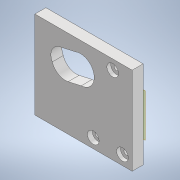
# Autodesk Inventor part: BOWDEN MOUNT
Saved by Autodesk Inventor 2020 (Build 240168000, 168)
## iProperties
Created: 2019-06-20
Part Number: BOWDEN MOUNT
Material: Generic
Document SubType Name: Modeling
Designer: pepd9
Density: 1 g/cm^3
Appearance: Default
Author: pepd9
Autodesk Inventor part; units mm, degrees
ref_plane "YZ Plane" through (0, 0, 0) normal (1, 0, 0) x (0, 1, 0)
ref_plane "XZ Plane" through (0, 0, 0) normal (0, 1, 0) x (-1, 0, 0)
ref_plane "XY Plane" through (0, 0, 0) normal (0, 0, 1) x (1, 0, 0)
ref_plane "Work Plane2" through (0, 0, 0) normal (0, 0, 1) x (1, 0, 0)
sketch "Sketch1" plane through (0, 0, 0) normal (0, 0, 1) x (1, 0, 0)
  line L0 (-10, 22.5) -> (10, 22.5)
  line L1 (10, 22.5) -> (10, -22.5)
  line L2 (10, -22.5) -> (-10, -22.5)
  line L3 (-10, -22.5) -> (-10, 22.5)
  circle A0 centre (0, 17.5) radius 1.25
  circle A1 centre (5, -17.5) radius 1.25
  point P0 (0, 0)
  dimension "d38" = 20
  dimension "d39" = 45
  dimension "d40" = 2.5
  dimension "d41" = 2.5
  dimension "d42" = 10
  dimension "d43" = 5
  dimension "d44" = 5
  dimension "d45" = 5
  constraints: 8 end point, 2 centre point, 2 parallel, 1 horizontal, 1 perpendicular
  measures "d38" distance of L0.start L0.end
  measures "d39" distance of L2.end L0.start
  measures "d40" diameter of A0
  measures "d41" diameter of A1
  measures "d42" distance from line of L1 A0.centre
  measures "d43" distance from line of L0 A0.centre
  measures "d44" distance from line of L2 A1.centre
  measures "d45" distance from line of L1 A1.centre
extrude "Extrusion1" add sketch "Sketch1" along normal blind 3.65 contours L0 L1 L2 L3 | A0 | A1
sketch "Sketch2" plane through (-10, 118.2358, 3.65) normal (-1, 0, 0) x (0, 0, 1)
  line L0 (-3.65, -95.7358) -> (-3.65, -140.7358) projected
  line L1 (-3.65, -140.7358) -> (0, -140.7358) projected
  line L2 (0, -95.7358) -> (0, -140.7358) projected
  line L3 (-3.65, -95.7358) -> (0, -95.7358) projected
  point P0 (-3.65, -118.2358)
extrude "Extrusion2" add sketch "Sketch2" along normal blind 30
sketch "Sketch3" plane through (0, 0, 3.65) normal (0, 0, 1) x (1, 0, 0)
  line L0 (10, -22.5) -> (10, 22.5) projected
  line L1 (10, 22.5) -> (-40, 22.5) projected
  line L2 (-40, -22.5) -> (-40, 22.5) projected
  line L3 (10, -22.5) -> (-40, -22.5) projected
  circle A0 centre (0, 17.5) radius 3 construction
  circle A1 centre (5, -17.5) radius 3 construction
  point P0 (0, 0)
  dimension "d48" = 6
  dimension "d49" = 6
  constraints: 2 centre point
  measures "d48" diameter of A0
  measures "d49" diameter of A1
extrude "Extrusion3" add sketch "Sketch3" along normal blind 2
ref_plane "Work Plane3" through (0, 0, 0) normal (0, 0, -1) x (-1, 0, 0)
sketch "Sketch10" plane through (0, 0, 5.65) normal (0, 0, 1) x (1, 0, 0)
  circle A0 centre (-10, -17.5) radius 2.5953
  line L0 (-40, -22.5) -> (10, -22.5) projected
  line L1 (10, -22.5) -> (10, 22.5) projected
  circle A1 centre (5, -17.5) radius 2.5953
  circle A2 centre (2, 17.5) radius 2.5953
  line L2 (10, 22.5) -> (-40, 22.5) projected
  point P0 (0, 0)
  dimension "d75" = 5
  dimension "d76" = 20
  dimension "d77" = 8
  dimension "d78" = 5
  dimension "d79" = 5
  dimension "d80" = 5
  constraints: 3 centre point
  measures "d75" distance from line of L0 A0.centre
  measures "d76" distance from line of L1 A0.centre
  measures "d77" distance from line of L1 A2.centre
  measures "d78" distance from line of L2 A2.centre
  measures "d79" distance from line of L1 A1.centre
  measures "d80" distance from line of A1.centre L0
hole "Hole4" at (-10, -17.5, 5.65) at (5, -17.5, 5.65) at (2, 17.5, 5.65) direction (0, 0, -1) diameter 3.1 end through all counterbore diameter 6 counterbore depth 1.9
body "Solid1"
